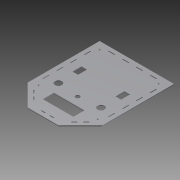
# Autodesk Inventor part: tutup kepala
Saved by Autodesk Inventor 2012 (Build 160160000, 160)
## iProperties
Created: 2013-12-07
Part Number: tutup kepala
Material: Default
Document SubType Name: Modeling
Designer: Irwan Haryanto
Density: 1 g/cm^3
Author: Irwan Haryanto
Autodesk Inventor part; units mm, degrees
ref_plane "YZ Plane" through (0, 0, 0) normal (1, 0, 0) x (0, 1, 0)
ref_plane "XZ Plane" through (0, 0, 0) normal (0, 1, 0) x (-1, 0, 0)
ref_plane "XY Plane" through (0, 0, 0) normal (0, 0, 1) x (1, 0, 0)
sketch "Sketch1" plane through (0, 0, 0) normal (0, 0, 1) x (1, 0, 0)
  line L0 (-77.4547, 22.5062) -> (-79.4547, 22.5062)
  line L1 (-88.4548, -106.3305) -> (-88.4548, 62.3216)
  line L2 (-77.4547, -10.4938) -> (-79.4547, -10.4938)
  line L3 (-77.4547, 4.5062) -> (-77.4547, -10.4938)
  line L4 (-79.4547, 4.5062) -> (-77.4547, 4.5062)
  line L5 (-79.4547, -10.4938) -> (-79.4547, 4.5062)
  line L6 (-77.4547, 37.5062) -> (-77.4547, 22.5062)
  line L7 (-79.4547, 37.5062) -> (-77.4547, 37.5062)
  line L8 (-79.4547, 22.5062) -> (-79.4547, 37.5062)
  line L9 (-77.4547, -42.4938) -> (-79.4547, -42.4938)
  line L10 (-77.4547, -27.4938) -> (-77.4547, -42.4938)
  line L11 (-79.4547, -42.4938) -> (-79.4547, -27.4938)
  line L12 (-79.4547, -27.4938) -> (-77.4547, -27.4938)
  line L13 (-58.1998, -33.3656) -> (-45.1998, -33.3656)
  line L14 (-45.1998, -33.3656) -> (-45.1998, -12.3656)
  line L15 (-58.1998, -12.3656) -> (-58.1998, -33.3656)
  line L16 (-45.1998, -12.3656) -> (-58.1998, -12.3656)
  line L17 (-79.4548, -60.4938) -> (-77.4548, -60.4938)
  line L18 (-77.4548, -60.4938) -> (-77.4548, -75.4938)
  line L19 (-79.4548, -75.4938) -> (-79.4548, -60.4938)
  line L20 (-77.4548, -75.4938) -> (-79.4548, -75.4938)
  circle A0 centre (-70.4548, -88.3305) radius 1.5
  line L21 (-57.6182, -95.3305) -> (-42.6182, -95.3305)
  line L22 (-42.6182, -95.3305) -> (-42.6182, -97.3305)
  line L23 (-42.6182, -97.3305) -> (-57.6182, -97.3305)
  line L24 (-57.6182, -97.3305) -> (-57.6182, -95.3305)
  line L25 (-65.7269, 69.4932) -> (-67.1411, 70.9074)
  line L26 (-60.0701, 77.9785) -> (-58.6558, 76.5643)
  line L27 (-58.6558, 76.5643) -> (-65.7269, 69.4932)
  line L28 (-67.1411, 70.9074) -> (-60.0701, 77.9785)
  line L29 (-45.9277, 92.1205) -> (-44.5135, 90.7062)
  line L30 (-44.5135, 90.7062) -> (-51.5846, 83.6352)
  line L31 (-52.9988, 85.0494) -> (-45.9277, 92.1205)
  line L32 (-88.4548, 62.3216) -> (-37.342, 113.4344)
  line L33 (-51.5846, 83.6352) -> (-52.9988, 85.0494)
  line L34 (-37.0998, 52.6344) -> (-37.0998, 78.4344)
  line L35 (-16.1999, 102.4344) -> (-16.1999, 104.4344)
  line L36 (-6.1999, 102.4344) -> (-16.1999, 102.4344)
  line L37 (-16.1999, 104.4344) -> (-6.1999, 104.4344)
  line L38 (-6.1999, 104.4344) -> (-6.1999, 102.4344)
  line L39 (3.8002, 102.4342) -> (3.8002, 104.4342)
  line L40 (13.8002, 102.4342) -> (3.8002, 102.4342)
  line L41 (13.8002, 104.4342) -> (13.8002, 102.4342)
  line L42 (3.8002, 104.4342) -> (13.8002, 104.4342)
  line L43 (-37.0998, 78.4344) -> (34.7002, 78.4344)
  line L44 (-37.342, 113.4344) -> (34.9424, 113.4344)
  line L45 (34.7002, 52.6344) -> (-37.0998, 52.6344)
  line L46 (34.7002, 78.4344) -> (34.7002, 52.6344)
  line L47 (22.3818, -95.3307) -> (22.3818, -97.3307)
  line L48 (40.3818, -97.3307) -> (40.3818, -95.3307)
  line L49 (55.3818, -95.3307) -> (55.3818, -97.3307)
  line L50 (55.3818, -97.3307) -> (40.3818, -97.3307)
  line L51 (40.3818, -95.3307) -> (55.3818, -95.3307)
  line L52 (7.3818, -95.3307) -> (22.3818, -95.3307)
  line L53 (22.3818, -97.3307) -> (7.3818, -97.3307)
  line L54 (7.3818, -97.3307) -> (7.3818, -95.3307)
  line L55 (86.0552, -106.3305) -> (-88.4548, -106.3305)
  line L56 (-9.6182, -95.3307) -> (-9.6182, -97.3307)
  line L57 (-24.6182, -95.3307) -> (-9.6182, -95.3307)
  line L58 (-24.6182, -97.3307) -> (-24.6182, -95.3307)
  line L59 (-9.6182, -97.3307) -> (-24.6182, -97.3307)
  line L60 (86.0552, 62.3216) -> (86.0552, -106.3305)
  circle A1 centre (68.0552, -88.3305) radius 1.5
  line L61 (75.0552, -75.4938) -> (77.0552, -75.4938)
  line L62 (77.0552, -60.4938) -> (75.0552, -60.4938)
  line L63 (77.0552, -75.4938) -> (77.0552, -60.4938)
  line L64 (75.055, -42.4938) -> (77.055, -42.4938)
  line L65 (75.055, -27.4938) -> (75.055, -42.4938)
  line L66 (77.055, -42.4938) -> (77.055, -27.4938)
  line L67 (75.0552, -60.4938) -> (75.0552, -75.4938)
  line L68 (42.8002, -12.3656) -> (55.8002, -12.3656)
  line L69 (77.055, 4.5062) -> (75.055, 4.5062)
  line L70 (75.055, 4.5062) -> (75.055, -10.4938)
  line L71 (77.055, -10.4938) -> (77.055, 4.5062)
  line L72 (42.8002, -33.3656) -> (42.8002, -12.3656)
  line L73 (75.055, -10.4938) -> (77.055, -10.4938)
  line L74 (55.8002, -12.3656) -> (55.8002, -33.3656)
  line L75 (55.8002, -33.3656) -> (42.8002, -33.3656)
  line L76 (77.055, -27.4938) -> (75.055, -27.4938)
  line L77 (77.055, 37.5062) -> (75.055, 37.5062)
  line L78 (75.055, 22.5062) -> (77.055, 22.5062)
  line L79 (77.055, 22.5062) -> (77.055, 37.5062)
  line L80 (75.055, 37.5062) -> (75.055, 22.5062)
  circle A2 centre (48.8002, 27.6344) radius 8
  circle A3 centre (68.0552, 54.8658) radius 1.5
  line L81 (64.6739, 70.8372) -> (63.2567, 69.426)
  line L82 (63.2567, 69.426) -> (56.2003, 76.5117)
  line L83 (56.2003, 76.5117) -> (57.6175, 77.9229)
  line L84 (57.6175, 77.9229) -> (64.6739, 70.8372)
  line L85 (50.5611, 85.0087) -> (49.1439, 83.5974)
  line L86 (49.1439, 83.5974) -> (42.0875, 90.6831)
  line L87 (42.0875, 90.6831) -> (43.5047, 92.0944)
  line L88 (43.5047, 92.0944) -> (50.5611, 85.0087)
  line L89 (34.9424, 113.4344) -> (86.0552, 62.3216)
  circle A4 centre (-70.4548, 54.8658) radius 1.5
  circle A5 centre (-51.1998, 27.6344) radius 8
  circle A6 centre (-1.1998, 32.6344) radius 4.85
  point P0 (0, 0)
  dimension "d44" = 10
  dimension "d45" = 2
  dimension "d46" = 10
  dimension "d47" = 2
  dimension "d48" = 10
  dimension "d49" = 2
  dimension "d50" = 10
  dimension "d51" = 2
  dimension "d52" = 10
  dimension "d53" = 10
  dimension "d54" = 2
  dimension "d55" = 10
  dimension "d56" = 2
  dimension "d57" = 10
  dimension "d58" = 15
  dimension "d59" = 2
  dimension "d60" = 15
  dimension "d61" = 18
  dimension "d62" = 15
  dimension "d63" = 17
  dimension "d64" = 2
  dimension "d65" = 15
  dimension "d66" = 15
  dimension "d67" = 18
  dimension "d68" = 15
  dimension "d69" = 17
  dimension "d70" = 15
  dimension "d71" = 18
  dimension "d72" = 15
  dimension "d73" = 18
  dimension "d74" = 219.7649
  dimension "d75" = 174.51
  dimension "d76" = 3
  dimension "d77" = 3
  dimension "d78" = 71.8
  dimension "d79" = 25.8
  dimension "d80" = 35
  dimension "d81" = 16
  dimension "d82" = 25
  dimension "d83" = 13
  dimension "d84" = 21
  dimension "d85" = 40
  dimension "d86" = 9.7
  dimension "d87" = 20
  constraints: 180 end point, 33 parallel, 17 perpendicular, 12 horizontal, 7 centre point
  measures "d44" distance of L36.start L35.start
  measures "d45" distance of L37.end L36.start
  measures "d46" distance of L40.start L39.start
  measures "d47" distance of L41.start L40.start
  measures "d48" distance of L26.end L27.end
  measures "d49" distance of L26.start L26.end
  measures "d50" distance of L29.end L30.end
  measures "d51" distance of L29.start L29.end
  measures "d52" distance between parallel lines of L33 L26
  measures "d53" distance of L85.end L87.start
  measures "d54" distance of L85.start L85.end
  measures "d55" distance of L81.end L82.end
  measures "d56" distance of L81.start L81.end
  measures "d57" distance between parallel lines of L83 L85
  measures "d58" distance of L22.end L23.end
  measures "d59" distance of L22.start L22.end
  measures "d60" distance of L56.end L58.start
  measures "d61" distance between parallel lines of L58 L22
  measures "d62" distance of L53.start L54.start
  measures "d63" distance between parallel lines of L54 L56
  measures "d64" distance of L18.end L19.start
  measures "d65" distance of L18.start L18.end
  measures "d66" distance of L12.end L10.end
  measures "d67" distance between parallel lines of L17 L9
  measures "d68" distance of L4.end L2.start
  measures "d69" distance between parallel lines of L12 L2
  measures "d70" distance of L6.start L0.start
  measures "d71" distance between parallel lines of L0 L4
  measures "d72" distance between parallel lines of L49 L48
  measures "d73" distance between parallel lines of L48 L47
  measures "d74" distance between parallel lines of L55 L44
  measures "d75" distance between parallel lines of L60 L1
  measures "d76" diameter of A3
  measures "d77" diameter of A1
  measures "d78" distance of L46.end L34.start
  measures "d79" distance of L46.start L46.end
  measures "d80" distance between parallel lines of L43 L44
  measures "d81" diameter of A2
  measures "d82" distance from line of L45 A2.centre
  measures "d83" distance of L75.start L75.end
  measures "d84" distance of L68.end L75.start
  measures "d85" distance from line of L68 A2.centre
  measures "d86" diameter of A6
  measures "d87" distance from line of A6.centre L45
extrude "Extrusion1" add sketch "Sketch1" along normal blind 2 contours L1 L32 L44 L89 L60 L55 | A0 | A1 | A3 | A4
sketch "Sketch2" plane through (0, 0, 2) normal (0, 0, 1) x (1, 0, 0)
  line L0 (-77.4547, -10.4938) -> (-79.4547, -10.4938)
  line L1 (-45.1998, -12.3656) -> (-58.1998, -12.3656)
  line L2 (-79.4547, 4.5062) -> (-77.4547, 4.5062)
  line L3 (-77.4547, 4.5062) -> (-77.4547, -10.4938)
  line L4 (-79.4547, -10.4938) -> (-79.4547, 4.5062)
  line L5 (-77.4547, 22.5062) -> (-79.4547, 22.5062)
  line L6 (-24.6182, -97.3307) -> (-24.6182, -95.3307)
  line L7 (-9.6182, -95.3307) -> (-9.6182, -97.3307)
  line L8 (-24.6182, -95.3307) -> (-9.6182, -95.3307)
  line L9 (-9.6182, -97.3307) -> (-24.6182, -97.3307)
  line L10 (-45.9277, 92.1205) -> (-44.5135, 90.7062)
  line L11 (-44.5135, 90.7062) -> (-51.5846, 83.6352)
  line L12 (-52.9988, 85.0494) -> (-45.9277, 92.1205)
  line L13 (-51.5846, 83.6352) -> (-52.9988, 85.0494)
  line L14 (-60.0701, 77.9785) -> (-58.6558, 76.5643)
  line L15 (-58.6558, 76.5643) -> (-65.7269, 69.4932)
  line L16 (-67.1411, 70.9074) -> (-60.0701, 77.9785)
  line L17 (-65.7269, 69.4932) -> (-67.1411, 70.9074)
  line L18 (-88.4548, 62.3216) -> (-37.342, 113.4344)
  line L19 (-88.4548, -106.3305) -> (-88.4548, 62.3216)
  line L20 (-58.1998, -12.3656) -> (-58.1998, -33.3656)
  line L21 (-45.1998, -33.3656) -> (-45.1998, -12.3656)
  line L22 (-79.4547, -27.4938) -> (-77.4547, -27.4938)
  line L23 (-58.1998, -33.3656) -> (-45.1998, -33.3656)
  line L24 (-79.4547, -42.4938) -> (-79.4547, -27.4938)
  line L25 (-77.4547, -27.4938) -> (-77.4547, -42.4938)
  line L26 (-77.4547, -42.4938) -> (-79.4547, -42.4938)
  line L27 (7.3818, -97.3307) -> (7.3818, -95.3307)
  line L28 (7.3818, -95.3307) -> (22.3818, -95.3307)
  line L29 (22.3818, -97.3307) -> (7.3818, -97.3307)
  line L30 (40.3818, -97.3307) -> (40.3818, -95.3307)
  line L31 (55.3818, -95.3307) -> (55.3818, -97.3307)
  line L32 (22.3818, -95.3307) -> (22.3818, -97.3307)
  line L33 (-16.1999, 102.4344) -> (-16.1999, 104.4344)
  line L34 (-6.1999, 102.4344) -> (-16.1999, 102.4344)
  line L35 (-16.1999, 104.4344) -> (-6.1999, 104.4344)
  line L36 (-6.1999, 104.4344) -> (-6.1999, 102.4344)
  line L37 (3.8002, 102.4342) -> (3.8002, 104.4342)
  line L38 (13.8002, 102.4342) -> (3.8002, 102.4342)
  line L39 (13.8002, 104.4342) -> (13.8002, 102.4342)
  line L40 (3.8002, 104.4342) -> (13.8002, 104.4342)
  circle A0 centre (-1.1998, 32.6344) radius 4.85
  line L41 (42.0875, 90.6831) -> (43.5047, 92.0944)
  line L42 (-37.0998, 52.6344) -> (-37.0998, 78.4344)
  line L43 (34.7002, 78.4344) -> (34.7002, 52.6344)
  line L44 (34.7002, 52.6344) -> (-37.0998, 52.6344)
  line L45 (-37.0998, 78.4344) -> (34.7002, 78.4344)
  line L46 (-37.342, 113.4344) -> (34.9424, 113.4344)
  line L47 (86.0552, -106.3305) -> (-88.4548, -106.3305)
  line L48 (-42.6182, -95.3305) -> (-42.6182, -97.3305)
  line L49 (-42.6182, -97.3305) -> (-57.6182, -97.3305)
  line L50 (-57.6182, -95.3305) -> (-42.6182, -95.3305)
  line L51 (-57.6182, -97.3305) -> (-57.6182, -95.3305)
  circle A1 centre (-70.4548, -88.3305) radius 1.5
  line L52 (-77.4548, -60.4938) -> (-77.4548, -75.4938)
  line L53 (-79.4548, -60.4938) -> (-77.4548, -60.4938)
  line L54 (-79.4548, -75.4938) -> (-79.4548, -60.4938)
  line L55 (-77.4548, -75.4938) -> (-79.4548, -75.4938)
  line L56 (55.3818, -97.3307) -> (40.3818, -97.3307)
  line L57 (40.3818, -95.3307) -> (55.3818, -95.3307)
  circle A2 centre (68.0552, -88.3305) radius 1.5
  line L58 (75.0552, -60.4938) -> (75.0552, -75.4938)
  line L59 (77.0552, -60.4938) -> (75.0552, -60.4938)
  line L60 (77.0552, -75.4938) -> (77.0552, -60.4938)
  line L61 (86.0552, 62.3216) -> (86.0552, -106.3305)
  line L62 (75.055, -42.4938) -> (77.055, -42.4938)
  line L63 (75.0552, -75.4938) -> (77.0552, -75.4938)
  line L64 (75.055, -27.4938) -> (75.055, -42.4938)
  line L65 (77.055, -42.4938) -> (77.055, -27.4938)
  line L66 (77.055, -27.4938) -> (75.055, -27.4938)
  line L67 (55.8002, -33.3656) -> (42.8002, -33.3656)
  line L68 (75.055, -10.4938) -> (77.055, -10.4938)
  line L69 (42.8002, -12.3656) -> (55.8002, -12.3656)
  line L70 (42.8002, -33.3656) -> (42.8002, -12.3656)
  line L71 (77.055, -10.4938) -> (77.055, 4.5062)
  line L72 (77.055, 4.5062) -> (75.055, 4.5062)
  line L73 (75.055, 4.5062) -> (75.055, -10.4938)
  line L74 (55.8002, -12.3656) -> (55.8002, -33.3656)
  line L75 (64.6739, 70.8372) -> (63.2567, 69.426)
  line L76 (63.2567, 69.426) -> (56.2003, 76.5117)
  line L77 (56.2003, 76.5117) -> (57.6175, 77.9229)
  line L78 (57.6175, 77.9229) -> (64.6739, 70.8372)
  line L79 (50.5611, 85.0087) -> (49.1439, 83.5974)
  line L80 (49.1439, 83.5974) -> (42.0875, 90.6831)
  line L81 (43.5047, 92.0944) -> (50.5611, 85.0087)
  line L82 (34.9424, 113.4344) -> (86.0552, 62.3216)
  line L83 (75.055, 22.5062) -> (77.055, 22.5062)
  line L84 (77.055, 37.5062) -> (75.055, 37.5062)
  line L85 (77.055, 22.5062) -> (77.055, 37.5062)
  line L86 (75.055, 37.5062) -> (75.055, 22.5062)
  circle A3 centre (68.0552, 54.8658) radius 1.5
  circle A4 centre (48.8002, 27.6344) radius 8
  circle A5 centre (-51.1998, 27.6344) radius 8
  line L87 (-77.4547, 37.5062) -> (-77.4547, 22.5062)
  line L88 (-79.4547, 22.5062) -> (-79.4547, 37.5062)
  line L89 (-79.4547, 37.5062) -> (-77.4547, 37.5062)
  circle A6 centre (-70.4548, 54.8658) radius 1.5
  point P0 (0, 0)
  point P1 (0, 0)
  dimension "d90" = 10
  dimension "d91" = 2
  dimension "d92" = 10
  dimension "d93" = 2
  dimension "d94" = 10
  dimension "d95" = 2
  dimension "d96" = 10
  dimension "d97" = 2
  dimension "d98" = 10
  dimension "d99" = 10
  dimension "d100" = 2
  dimension "d101" = 10
  dimension "d102" = 2
  dimension "d103" = 10
  dimension "d104" = 15
  dimension "d105" = 2
  dimension "d106" = 15
  dimension "d107" = 18
  dimension "d108" = 15
  dimension "d109" = 17
  dimension "d110" = 2
  dimension "d111" = 15
  dimension "d112" = 15
  dimension "d113" = 18
  dimension "d114" = 15
  dimension "d115" = 17
  dimension "d116" = 15
  dimension "d117" = 18
  dimension "d118" = 15
  dimension "d119" = 18
  dimension "d120" = 219.7649
  dimension "d121" = 174.51
  dimension "d122" = 3
  dimension "d123" = 3
  dimension "d124" = 71.8
  dimension "d125" = 25.8
  dimension "d126" = 35
  dimension "d127" = 16
  dimension "d128" = 25
  dimension "d129" = 13
  dimension "d130" = 21
  dimension "d131" = 40
  dimension "d132" = 9.7
  dimension "d133" = 20
  constraints: 180 end point, 33 parallel, 17 perpendicular, 12 horizontal, 7 centre point
  measures "d90" distance of L34.start L33.start
  measures "d91" distance of L35.end L34.start
  measures "d92" distance of L38.start L38.end
  measures "d93" distance of L39.start L38.start
  measures "d94" distance of L14.end L15.end
  measures "d95" distance of L14.start L14.end
  measures "d96" distance of L10.end L11.end
  measures "d97" distance of L10.start L10.end
  measures "d98" distance between parallel lines of L13 L14
  measures "d99" distance of L79.end L41.start
  measures "d100" distance of L79.start L79.end
  measures "d101" distance of L75.end L76.end
  measures "d102" distance of L75.start L75.end
  measures "d103" distance between parallel lines of L77 L79
  measures "d104" distance of L48.end L49.end
  measures "d105" distance of L48.start L48.end
  measures "d106" distance of L7.end L9.end
  measures "d107" distance between parallel lines of L6 L48
  measures "d108" distance of L29.start L27.start
  measures "d109" distance between parallel lines of L27 L7
  measures "d110" distance of L55.start L55.end
  measures "d111" distance of L52.start L55.start
  measures "d112" distance of L22.end L25.end
  measures "d113" distance between parallel lines of L53 L26
  measures "d114" distance of L2.end L0.start
  measures "d115" distance between parallel lines of L22 L0
  measures "d116" distance of L89.end L5.start
  measures "d117" distance between parallel lines of L5 L2
  measures "d118" distance between parallel lines of L31 L30
  measures "d119" distance between parallel lines of L30 L32
  measures "d120" distance between parallel lines of L47 L46
  measures "d121" distance between parallel lines of L61 L19
  measures "d122" diameter of A3
  measures "d123" diameter of A2
  measures "d124" distance of L44.start L44.end
  measures "d125" distance of L45.end L44.start
  measures "d126" distance between parallel lines of L45 L46
  measures "d127" diameter of A4
  measures "d128" distance from line of L44 A4.centre
  measures "d129" distance of L74.end L70.start
  measures "d130" distance of L74.start L74.end
  measures "d131" distance from line of L69 A4.centre
  measures "d132" diameter of A0
  measures "d133" distance from line of A0.centre L44
hole "Hole1" at (-70.4548, 54.8658, 2) at (68.0552, 54.8658, 2) at (68.0552, -88.3305, 2) at (-70.4548, -88.3305, 2) direction (0, 0, -1) diameter 3 end through all
body "Solid1"
